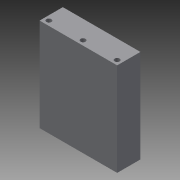
# Autodesk Inventor part: brush rack
Saved by Autodesk Inventor 2013 SP2 (Build 170200200, 200)
## iProperties
Created: 2017-05-30
Part Number: brush rack
Material: Generic
Document SubType Name: Modeling
Designer: Herman de Vries
Density: 1 g/cm^3
Author: Herman de Vries
Autodesk Inventor part; units mm, degrees
ref_plane "YZ Plane" through (0, 0, 0) normal (1, 0, 0) x (0, 1, 0)
ref_plane "XZ Plane" through (0, 0, 0) normal (0, 1, 0) x (-1, 0, 0)
ref_plane "XY Plane" through (0, 0, 0) normal (0, 0, 1) x (1, 0, 0)
sketch "Sketch1" plane through (0, 0, 0) normal (0, 0, 1) x (1, 0, 0)
  line L0 (0, 0) -> (50, 0)
  line L1 (50, 0) -> (50, 15)
  line L2 (50, 15) -> (0, 15)
  line L3 (0, 15) -> (0, 0)
  dimension "d0" = 50
  dimension "d1" = 15
  constraints: 8 end point, 2 parallel, 1 horizontal, 1 perpendicular
  measures "d0" distance of L2.end L1.end
  measures "d1" distance of L1.end L0.end
extrude "Extrusion1" add sketch "Sketch1" along normal blind 60
sketch "Sketch2" plane through (0, 0, 60) normal (0, 0, 1) x (1, 0, 0)
  circle A0 centre (3, 3) radius 1.6
  circle A1 centre (47, 3) radius 1.6
  circle A2 centre (25, 3) radius 1.6
  line L0 (0, 15) -> (0, 0) projected
  line L1 (50, 0) -> (50, 15) projected
  line L2 (0, 0) -> (50, 0) projected
  point P0 (25, 0)
  dimension "d4" = 3.2
  dimension "d5" = 3.2
  dimension "d6" = 3.2
  dimension "d7" = 3
  dimension "d8" = 3
  dimension "d11" = 3
  constraints: 3 centre point, 2 horizontal alignment, 1 midpoint, 1 vertical alignment
  measures "d4" diameter of A0
  measures "d5" diameter of A1
  measures "d6" diameter of A2
  measures "d7" distance from line of A0.centre L0
  measures "d8" distance from line of A1.centre L1
  measures "d11" horizontal distance of L0.end A0.centre
extrude "Extrusion2" cut sketch "Sketch2" against normal blind 10
body "Solid1"
